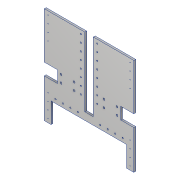
# Autodesk Inventor part: Piv Pannel
Saved by Autodesk Inventor 2018 (Build 220112000, 112)
## iProperties
Created: 2018-01-09
Part Number: Piv Pannel
Material: Aluminum 6061
Document SubType Name: Modeling
Designer: dsayers
Density: 2.7 g/cm^3
Appearance: Aluminum - Flat
Mass: 1658.47 g
Surface Area: 2042.47 cm^2
Volume: 614.249 cm^3
Author: dsayers
Autodesk Inventor part; units mm, degrees
ref_plane "YZ Plane" through (0, 0, 0) normal (1, 0, 0) x (0, 1, 0)
ref_plane "XZ Plane" through (0, 0, 0) normal (0, 1, 0) x (-1, 0, 0)
ref_plane "XY Plane" through (0, 0, 0) normal (0, 0, 1) x (1, 0, 0)
sketch "Sketch1" plane through (0, 0, 0) normal (0, 0, 1) x (1, 0, 0)
  line L0 (0, 0) -> (304.8, 0)
  line L1 (304.8, 0) -> (304.8, 330.2)
  line L2 (304.8, 330.2) -> (0, 330.2)
  line L3 (0, 330.2) -> (0, 0)
  dimension "d0" = 304.8
  dimension "d1" = 330.2
  constraints: 8 end point, 2 parallel, 1 horizontal, 1 perpendicular
  measures "d0" distance of L1.end L2.end
  measures "d1" distance of L0.end L1.end
extrude "Extrusion1" add sketch "Sketch1" along normal blind 6.35
sketch "Sketch2" plane through (0, 0, 6.35) normal (0, 0, 1) x (1, 0, 0)
  circle A0 centre (57.0998, 139.7) radius 3.175 projected
  circle A1 centre (101.5498, 165.1) radius 3.175 projected
  circle A2 centre (203.2502, 139.7) radius 3.175 projected
  circle A3 centre (247.7002, 165.1) radius 3.175 projected
  circle A4 centre (203.2502, 165.1) radius 3.175 projected
  circle A5 centre (247.7002, 139.7) radius 3.175 projected
  circle A6 centre (101.5498, 139.7) radius 3.175 projected
  circle A7 centre (57.0998, 165.1) radius 3.175 projected
  line L0 (0, 132.2) -> (44.7998, 132.2) projected
  line L1 (44.7998, 132.2) -> (44.7998, 172.6) projected
  line L2 (44.7998, 172.6) -> (0, 172.6) projected
  line L3 (0, 330.2) -> (0, 172.6) projected
  line L4 (304.8, 330.2) -> (0, 330.2) projected
  line L5 (304.8, 172.6) -> (304.8, 330.2) projected
  line L6 (304.8, 172.6) -> (260.0002, 172.6) projected
  line L7 (260.0002, 172.6) -> (260.0002, 132.2) projected
  line L8 (260.0002, 132.2) -> (304.8, 132.2) projected
  line L9 (304.8, 120.65) -> (304.8, 132.2) projected
  line L10 (0, 0) -> (22.86, 0) projected
  line L11 (0, 132.2) -> (0, 0) projected
  line L12 (44.7998, 172.6) -> (0, 172.6)
  line L13 (0, 172.6) -> (0, 132.2)
  line L14 (0, 132.2) -> (44.7998, 132.2)
  line L15 (44.7998, 132.2) -> (44.7998, 172.6)
  line L16 (260.0002, 172.6) -> (304.8, 172.6)
  line L17 (304.8, 172.6) -> (304.8, 132.2)
  line L18 (304.8, 132.2) -> (260.0002, 132.2)
  line L19 (260.0002, 132.2) -> (260.0002, 172.6)
  circle A8 centre (12.7, 38.1) radius 0.889 projected
  circle A9 centre (12.7, 88.9) radius 0.889 projected
  circle A10 centre (12.7, 266.7) radius 0.889 projected
  circle A11 centre (12.7, 317.5) radius 0.889 projected
  circle A12 centre (12.7, 292.1) radius 0.889 projected
  circle A13 centre (12.7, 241.3) radius 0.889 projected
  circle A14 centre (12.7, 63.5) radius 0.889 projected
  circle A15 centre (12.7, 12.7) radius 0.889 projected
  circle A16 centre (292.1, 266.7) radius 0.889 projected
  circle A17 centre (292.1, 317.5) radius 0.889 projected
  circle A18 centre (292.1, 292.1) radius 0.889 projected
  circle A19 centre (292.1, 241.3) radius 0.889 projected
  circle A20 centre (124.5248, 317.5) radius 2.2479 projected
  circle A21 centre (124.5248, 292.1) radius 2.2479 projected
  circle A22 centre (180.2752, 266.7) radius 2.2479 projected
  circle A23 centre (124.5248, 241.3) radius 2.2479 projected
  circle A24 centre (124.5248, 215.9) radius 2.2479 projected
  circle A25 centre (180.2752, 190.5) radius 2.2479 projected
  circle A26 centre (124.5248, 165.1) radius 2.2479 projected
  circle A27 centre (180.2752, 139.7) radius 2.2479 projected
  circle A28 centre (124.5248, 139.7) radius 2.2479 projected
  circle A29 centre (180.2752, 165.1) radius 2.2479 projected
  circle A30 centre (124.5248, 190.5) radius 2.2479 projected
  circle A31 centre (180.2752, 215.9) radius 2.2479 projected
  circle A32 centre (180.2752, 241.3) radius 2.2479 projected
  circle A33 centre (124.5248, 266.7) radius 2.2479 projected
  circle A34 centre (180.2752, 292.1) radius 2.2479 projected
  circle A35 centre (180.2752, 317.5) radius 2.2479 projected
  line L20 (167.5752, 120.65) -> (167.5752, 215.9) projected
  line L21 (167.5752, 215.9) -> (137.2248, 215.9) projected
  line L22 (137.2248, 215.9) -> (137.2248, 120.65) projected
  line L23 (22.86, 120.65) -> (22.86, 0) projected
  line L24 (304.8, 120.65) -> (167.5752, 120.65) projected
  line L25 (137.2248, 120.65) -> (22.86, 120.65) projected
  constraints: 16 end point, 4 parallel, 2 horizontal, 2 perpendicular
extrude "Extrusion2" cut sketch "Sketch2" against normal blind 6.35 contours L13 L2 L1 L0 | L17 L8 L7 L6
sketch "Sketch3" plane through (0, 0, 6.35) normal (0, 0, 1) x (1, 0, 0)
  circle A0 centre (57.0998, 139.7) radius 3.175 projected
  circle A1 centre (101.5498, 165.1) radius 3.175 projected
  circle A2 centre (203.2502, 139.7) radius 3.175 projected
  circle A3 centre (247.7002, 165.1) radius 3.175 projected
  circle A4 centre (203.2502, 165.1) radius 3.175 projected
  circle A5 centre (247.7002, 139.7) radius 3.175 projected
  circle A6 centre (101.5498, 139.7) radius 3.175 projected
  circle A7 centre (57.0998, 165.1) radius 3.175 projected
  line L0 (0, 132.2) -> (44.7998, 132.2) projected
  line L1 (44.7998, 132.2) -> (44.7998, 172.6) projected
  line L2 (44.7998, 172.6) -> (0, 172.6) projected
  line L3 (0, 330.2) -> (0, 172.6) projected
  line L4 (304.8, 330.2) -> (0, 330.2) projected
  line L5 (304.8, 172.6) -> (304.8, 330.2) projected
  line L6 (304.8, 172.6) -> (260.0002, 172.6) projected
  line L7 (260.0002, 172.6) -> (260.0002, 132.2) projected
  line L8 (260.0002, 132.2) -> (304.8, 132.2) projected
  line L9 (304.8, 120.65) -> (304.8, 132.2) projected
  line L10 (0, 0) -> (22.86, 0) projected
  line L11 (0, 132.2) -> (0, 0) projected
  circle A8 centre (12.7, 38.1) radius 0.889 projected
  circle A9 centre (12.7, 88.9) radius 0.889 projected
  circle A10 centre (12.7, 266.7) radius 0.889 projected
  circle A11 centre (12.7, 317.5) radius 0.889 projected
  circle A12 centre (12.7, 292.1) radius 0.889 projected
  circle A13 centre (12.7, 241.3) radius 0.889 projected
  circle A14 centre (12.7, 63.5) radius 0.889 projected
  circle A15 centre (12.7, 12.7) radius 0.889 projected
  circle A16 centre (292.1, 266.7) radius 0.889 projected
  circle A17 centre (292.1, 317.5) radius 0.889 projected
  circle A18 centre (292.1, 292.1) radius 0.889 projected
  circle A19 centre (292.1, 241.3) radius 0.889 projected
  circle A20 centre (124.5248, 317.5) radius 2.2479 projected
  circle A21 centre (124.5248, 292.1) radius 2.2479 projected
  circle A22 centre (180.2752, 266.7) radius 2.2479 projected
  circle A23 centre (124.5248, 241.3) radius 2.2479 projected
  circle A24 centre (124.5248, 215.9) radius 2.2479 projected
  circle A25 centre (180.2752, 190.5) radius 2.2479 projected
  circle A26 centre (124.5248, 165.1) radius 2.2479 projected
  circle A27 centre (180.2752, 139.7) radius 2.2479 projected
  circle A28 centre (124.5248, 139.7) radius 2.2479 projected
  circle A29 centre (180.2752, 165.1) radius 2.2479 projected
  circle A30 centre (124.5248, 190.5) radius 2.2479 projected
  circle A31 centre (180.2752, 215.9) radius 2.2479 projected
  circle A32 centre (180.2752, 241.3) radius 2.2479 projected
  circle A33 centre (124.5248, 266.7) radius 2.2479 projected
  circle A34 centre (180.2752, 292.1) radius 2.2479 projected
  circle A35 centre (180.2752, 317.5) radius 2.2479 projected
  line L12 (167.5752, 120.65) -> (167.5752, 215.9) projected
  line L13 (167.5752, 215.9) -> (137.2248, 215.9) projected
  line L14 (137.2248, 215.9) -> (137.2248, 120.65) projected
  line L15 (22.86, 120.65) -> (22.86, 0) projected
  line L16 (304.8, 120.65) -> (167.5752, 120.65) projected
  line L17 (137.2248, 120.65) -> (22.86, 120.65) projected
  point P0 (57.0998, 165.1)
  point P1 (57.0998, 139.7)
  point P2 (101.5498, 139.7)
  point P3 (101.5498, 165.1)
  point P4 (203.2502, 165.1)
  point P5 (203.2502, 139.7)
  point P6 (247.7002, 139.7)
  point P7 (247.7002, 165.1)
  constraints: 8 coincident
hole "Hole1" at (57.0998, 165.1, 6.35) at (57.0998, 139.7, 6.35) at (101.5498, 139.7, 6.35) at (101.5498, 165.1, 6.35) at (203.2502, 165.1, 6.35) at (203.2502, 139.7, 6.35) at (247.7002, 139.7, 6.35) at (247.7002, 165.1, 6.35) direction (0, 0, -1) diameter 6.35 depth 25.4 tip angle 118
sketch "Sketch4" plane through (0, 0, 6.35) normal (0, 0, 1) x (1, 0, 0)
  circle A0 centre (12.7, 38.1) radius 0.889 projected
  circle A1 centre (12.7, 88.9) radius 0.889 projected
  circle A2 centre (12.7, 266.7) radius 0.889 projected
  circle A3 centre (12.7, 317.5) radius 0.889 projected
  circle A4 centre (12.7, 292.1) radius 0.889 projected
  circle A5 centre (12.7, 241.3) radius 0.889 projected
  circle A6 centre (12.7, 63.5) radius 0.889 projected
  circle A7 centre (12.7, 12.7) radius 0.889 projected
  circle A8 centre (292.1, 266.7) radius 0.889 projected
  circle A9 centre (292.1, 317.5) radius 0.889 projected
  circle A10 centre (292.1, 292.1) radius 0.889 projected
  circle A11 centre (292.1, 241.3) radius 0.889 projected
  circle A12 centre (57.0998, 139.7) radius 3.175 projected
  circle A13 centre (101.5498, 165.1) radius 3.175 projected
  circle A14 centre (203.2502, 139.7) radius 3.175 projected
  circle A15 centre (247.7002, 165.1) radius 3.175 projected
  circle A16 centre (203.2502, 165.1) radius 3.175 projected
  circle A17 centre (247.7002, 139.7) radius 3.175 projected
  circle A18 centre (101.5498, 139.7) radius 3.175 projected
  circle A19 centre (57.0998, 165.1) radius 3.175 projected
  line L0 (0, 132.2) -> (44.7998, 132.2) projected
  line L1 (44.7998, 132.2) -> (44.7998, 172.6) projected
  line L2 (44.7998, 172.6) -> (0, 172.6) projected
  line L3 (0, 330.2) -> (0, 172.6) projected
  line L4 (304.8, 330.2) -> (0, 330.2) projected
  line L5 (304.8, 172.6) -> (304.8, 330.2) projected
  line L6 (304.8, 172.6) -> (260.0002, 172.6) projected
  line L7 (260.0002, 172.6) -> (260.0002, 132.2) projected
  line L8 (260.0002, 132.2) -> (304.8, 132.2) projected
  line L9 (304.8, 120.65) -> (304.8, 132.2) projected
  line L10 (0, 0) -> (22.86, 0) projected
  line L11 (0, 132.2) -> (0, 0) projected
  circle A20 centre (124.5248, 317.5) radius 2.2479 projected
  circle A21 centre (124.5248, 292.1) radius 2.2479 projected
  circle A22 centre (180.2752, 266.7) radius 2.2479 projected
  circle A23 centre (124.5248, 241.3) radius 2.2479 projected
  circle A24 centre (124.5248, 215.9) radius 2.2479 projected
  circle A25 centre (180.2752, 190.5) radius 2.2479 projected
  circle A26 centre (124.5248, 165.1) radius 2.2479 projected
  circle A27 centre (180.2752, 139.7) radius 2.2479 projected
  circle A28 centre (124.5248, 139.7) radius 2.2479 projected
  circle A29 centre (180.2752, 165.1) radius 2.2479 projected
  circle A30 centre (124.5248, 190.5) radius 2.2479 projected
  circle A31 centre (180.2752, 215.9) radius 2.2479 projected
  circle A32 centre (180.2752, 241.3) radius 2.2479 projected
  circle A33 centre (124.5248, 266.7) radius 2.2479 projected
  circle A34 centre (180.2752, 292.1) radius 2.2479 projected
  circle A35 centre (180.2752, 317.5) radius 2.2479 projected
  line L12 (167.5752, 120.65) -> (167.5752, 215.9) projected
  line L13 (167.5752, 215.9) -> (137.2248, 215.9) projected
  line L14 (137.2248, 215.9) -> (137.2248, 120.65) projected
  line L15 (22.86, 120.65) -> (22.86, 0) projected
  line L16 (304.8, 120.65) -> (167.5752, 120.65) projected
  line L17 (137.2248, 120.65) -> (22.86, 120.65) projected
  point P0 (12.7, 317.5)
  point P1 (12.7, 292.1)
  point P2 (12.7, 266.7)
  point P3 (12.7, 241.3)
  point P4 (12.7, 88.9)
  point P5 (292.1, 88.9)
  point P6 (292.1, 63.5)
  point P7 (292.1, 38.1)
  point P8 (292.1, 12.7)
  point P9 (292.1, 241.3)
  point P10 (292.1, 266.7)
  point P11 (292.1, 292.1)
  point P12 (292.1, 317.5)
  constraints: 12 coincident
hole "Hole2" at (12.7, 317.5, 6.35) at (12.7, 292.1, 6.35) at (12.7, 266.7, 6.35) at (12.7, 241.3, 6.35) at (12.7, 88.9, 6.35) at (12.7, 63.5, 6.35) at (12.7, 38.1, 6.35) at (12.7, 12.7, 6.35) at (292.1, 88.9, 6.35) at (292.1, 63.5, 6.35) at (292.1, 38.1, 6.35) at (292.1, 12.7, 6.35) at (292.1, 241.3, 6.35) at (292.1, 266.7, 6.35) at (292.1, 292.1, 6.35) at (292.1, 317.5, 6.35) direction (0, 0, -1) diameter 1.778 depth 25.4 tip angle 118 clearance for "Flat Head Machine Screw (82)" size "#0" standard "Ansi Unified Screw Threads"
sketch "Sketch5" plane through (0, 0, 6.35) normal (0, 0, 1) x (1, 0, 0)
  line L0 (165.1, 322.2478) -> (165.1, -126.1091) projected
  line L1 (139.7, 322.2478) -> (139.7, -126.1091) projected
  line L2 (139.7, 254) -> (165.1, 254)
  line L3 (165.1, 254) -> (165.1, 330.2)
  line L4 (165.1, 330.2) -> (139.7, 330.2)
  line L5 (139.7, 330.2) -> (139.7, 254)
  line L6 (304.8, 330.2) -> (0, 330.2) projected
  point P0 (0, 0)
  dimension "d20" = 0
  dimension "d21" = 76.2
  constraints: 8 end point, 2 parallel, 1 horizontal, 1 perpendicular, 1 point on line
  measures "d20" distance between parallel lines of L6 L4
  measures "d21" distance between parallel lines of L6 L2
extrude "Extrusion3" cut sketch "Sketch5" against normal blind 6.35
sketch "Sketch6" plane through (0, 0, 6.35) normal (0, 0, 1) x (1, 0, 0)
  line L0 (304.8, 330.2) -> (165.1, 330.2) projected
  line L1 (165.1, 330.2) -> (166.6875, 330.2)
  line L2 (166.6875, 330.2) -> (166.6875, 254)
  line L3 (166.6875, 254) -> (165.1, 254)
  line L4 (165.1, 254) -> (165.1, 330.2)
  line L5 (139.7, 330.2) -> (0, 330.2) projected
  line L6 (139.7, 330.2) -> (138.1125, 330.2)
  line L7 (138.1125, 330.2) -> (138.1125, 254)
  line L8 (138.1125, 254) -> (139.7, 254)
  line L9 (139.7, 254) -> (139.7, 330.2)
  line L10 (139.7, 254) -> (139.7, 330.2) projected
  point P0 (0, 0)
  dimension "d24" = 1.5875
  dimension "d25" = 1.5875
  constraints: 16 end point, 4 parallel, 2 horizontal, 2 perpendicular
  measures "d24" distance of L2.end L3.end
  measures "d25" distance between parallel lines of L10 L7
extrude "Extrusion4" cut sketch "Sketch6" against normal blind 6.35
sketch "Sketch7" plane through (0, 0, 6.35) normal (0, 0, 1) x (1, 0, 0)
  line L0 (142.24, 177.7506) -> (142.24, -148.2697) projected
  line L1 (165.1, 175.9057) -> (165.1, -141.7236) projected
  line L2 (139.7, 128.8943) -> (139.7, -188.735) projected
  line L3 (165.1, 175.9057) -> (139.7, 175.9057)
  line L4 (139.7, 175.9057) -> (139.7, 95.25)
  line L5 (139.7, 95.25) -> (165.1, 95.25)
  line L6 (165.1, 95.25) -> (165.1, 175.9057)
  line L7 (0, 0) -> (304.8, 0) projected
  line L8 (139.7, 175.9057) -> (165.1, 175.9057)
  line L9 (165.1, 175.9057) -> (165.1, 196.85)
  line L10 (165.1, 196.85) -> (139.7, 196.85)
  line L11 (139.7, 196.85) -> (139.7, 175.9057)
  dimension "d28" = 95.25
  dimension "d29" = 0
  dimension "d30" = 101.6
  constraints: 16 end point, 4 parallel, 2 horizontal, 2 perpendicular, 1 point on line
  measures "d28" distance between parallel lines of L7 L5
  measures "d29" distance between parallel lines of L1 L9
  measures "d30" distance between parallel lines of L5 L10
extrude "Extrusion5" cut sketch "Sketch7" against normal blind 6.35 contours L3 L1 L5 L0 | L3 L11 L10 L9 | L0 L5 L2 L4 L3
sketch "Sketch8" plane through (0, 0, 6.35) normal (0, 0, 1) x (1, 0, 0)
  line L0 (138.1125, 330.2) -> (138.1125, 254) projected
  line L1 (138.1125, 330.2) -> (166.6875, 330.2)
  line L2 (166.6875, 330.2) -> (166.6875, 95.25)
  line L3 (166.6875, 95.25) -> (138.1125, 95.25)
  line L4 (138.1125, 95.25) -> (138.1125, 330.2)
  line L5 (166.6875, 330.2) -> (166.6875, 254) projected
  line L6 (165.1, 95.25) -> (139.7, 95.25) projected
  point P0 (0, 0)
  dimension "d33" = 0
  dimension "d34" = 0
  constraints: 8 end point, 2 parallel, 1 horizontal, 1 perpendicular
  measures "d33" distance between parallel lines of L5 L2
  measures "d34" distance between parallel lines of L6 L3
extrude "Extrusion6" cut sketch "Sketch8" against normal blind 6.35
sketch "Sketch10" plane through (0, 0, 6.35) normal (0, 0, 1) x (1, 0, 0)
  circle A0 centre (124.5248, 317.5) radius 2.2479 projected
  circle A1 centre (124.5248, 292.1) radius 2.2479 projected
  circle A2 centre (180.2752, 266.7) radius 2.2479 projected
  circle A3 centre (124.5248, 241.3) radius 2.2479 projected
  circle A4 centre (124.5248, 215.9) radius 2.2479 projected
  circle A5 centre (180.2752, 190.5) radius 2.2479 projected
  circle A6 centre (124.5248, 165.1) radius 2.2479 projected
  circle A7 centre (180.2752, 139.7) radius 2.2479 projected
  circle A8 centre (124.5248, 139.7) radius 2.2479 projected
  circle A9 centre (180.2752, 165.1) radius 2.2479 projected
  circle A10 centre (124.5248, 190.5) radius 2.2479 projected
  circle A11 centre (180.2752, 215.9) radius 2.2479 projected
  circle A12 centre (180.2752, 241.3) radius 2.2479 projected
  circle A13 centre (124.5248, 266.7) radius 2.2479 projected
  circle A14 centre (180.2752, 292.1) radius 2.2479 projected
  circle A15 centre (180.2752, 317.5) radius 2.2479 projected
  circle A16 centre (12.7, 38.1) radius 0.889 projected
  circle A17 centre (12.7, 88.9) radius 0.889 projected
  circle A18 centre (12.7, 266.7) radius 0.889 projected
  circle A19 centre (12.7, 317.5) radius 0.889 projected
  circle A20 centre (12.7, 292.1) radius 0.889 projected
  circle A21 centre (12.7, 241.3) radius 0.889 projected
  circle A22 centre (12.7, 63.5) radius 0.889 projected
  circle A23 centre (12.7, 12.7) radius 0.889 projected
  circle A24 centre (292.1, 266.7) radius 0.889 projected
  circle A25 centre (292.1, 317.5) radius 0.889 projected
  circle A26 centre (292.1, 292.1) radius 0.889 projected
  circle A27 centre (292.1, 241.3) radius 0.889 projected
  circle A28 centre (57.0998, 139.7) radius 3.175 projected
  circle A29 centre (101.5498, 165.1) radius 3.175 projected
  circle A30 centre (203.2502, 139.7) radius 3.175 projected
  circle A31 centre (247.7002, 165.1) radius 3.175 projected
  circle A32 centre (203.2502, 165.1) radius 3.175 projected
  circle A33 centre (247.7002, 139.7) radius 3.175 projected
  circle A34 centre (101.5498, 139.7) radius 3.175 projected
  circle A35 centre (57.0998, 165.1) radius 3.175 projected
  line L0 (0, 132.2) -> (44.7998, 132.2) projected
  line L1 (44.7998, 132.2) -> (44.7998, 172.6) projected
  line L2 (44.7998, 172.6) -> (0, 172.6) projected
  line L3 (0, 330.2) -> (0, 172.6) projected
  line L4 (304.8, 330.2) -> (0, 330.2) projected
  line L5 (304.8, 172.6) -> (304.8, 330.2) projected
  line L6 (304.8, 172.6) -> (260.0002, 172.6) projected
  line L7 (260.0002, 172.6) -> (260.0002, 132.2) projected
  line L8 (260.0002, 132.2) -> (304.8, 132.2) projected
  line L9 (304.8, 120.65) -> (304.8, 132.2) projected
  line L10 (0, 0) -> (22.86, 0) projected
  line L11 (0, 132.2) -> (0, 0) projected
  line L12 (167.5752, 120.65) -> (167.5752, 215.9) projected
  line L13 (167.5752, 215.9) -> (137.2248, 215.9) projected
  line L14 (137.2248, 215.9) -> (137.2248, 120.65) projected
  line L15 (22.86, 120.65) -> (22.86, 0) projected
  line L16 (304.8, 120.65) -> (167.5752, 120.65) projected
  line L17 (137.2248, 120.65) -> (22.86, 120.65) projected
  constraints: 16 coincident
hole "Hole3" at (124.5248, 317.5, 6.35) at (124.5248, 292.1, 6.35) at (124.5248, 266.7, 6.35) at (124.5248, 241.3, 6.35) at (124.5248, 215.9, 6.35) at (124.5248, 190.5, 6.35) at (124.5248, 165.1, 6.35) at (124.5248, 139.7, 6.35) at (180.2752, 139.7, 6.35) at (180.2752, 165.1, 6.35) at (180.2752, 190.5, 6.35) at (180.2752, 215.9, 6.35) at (180.2752, 241.3, 6.35) at (180.2752, 266.7, 6.35) at (180.2752, 292.1, 6.35) at (180.2752, 317.5, 6.35) direction (0, 0, -1) diameter 4.4958 depth 25.4 tip angle 118 clearance for "Flat Head Machine Screw (82)" size "#8" standard "Ansi Unified Screw Threads"
sketch "Sketch11" plane through (0, 0, 0) normal (0, 0, -1) x (-1, 0, 0)
  line L0 (-22.86, 120.65) -> (-22.86, 0) projected
  line L1 (0, 0) -> (-22.86, 0) projected
  line L2 (0, 132.2) -> (0, 0) projected
  line L3 (0, 132.2) -> (-44.7998, 132.2) projected
  line L4 (-44.7998, 132.2) -> (-44.7998, 172.6) projected
  line L5 (-44.7998, 172.6) -> (0, 172.6) projected
  line L6 (0, 330.2) -> (0, 172.6) projected
  line L7 (-304.8, 330.2) -> (0, 330.2) projected
  line L8 (-304.8, 172.6) -> (-304.8, 330.2) projected
  line L9 (-304.8, 172.6) -> (-260.0002, 172.6) projected
  line L10 (-260.0002, 172.6) -> (-260.0002, 132.2) projected
  line L11 (-260.0002, 132.2) -> (-304.8, 132.2) projected
  line L12 (-304.8, 120.65) -> (-304.8, 132.2) projected
  line L13 (-304.8, 120.65) -> (-167.5752, 120.65) projected
  line L14 (-167.5752, 120.65) -> (-167.5752, 215.9) projected
  line L15 (-167.5752, 215.9) -> (-137.2248, 215.9) projected
  line L16 (-137.2248, 215.9) -> (-137.2248, 120.65) projected
  circle A0 centre (-124.5248, 317.5) radius 2.2479 projected
  circle A1 centre (-124.5248, 292.1) radius 2.2479 projected
  circle A2 centre (-180.2752, 266.7) radius 2.2479 projected
  circle A3 centre (-124.5248, 241.3) radius 2.2479 projected
  circle A4 centre (-124.5248, 215.9) radius 2.2479 projected
  circle A5 centre (-180.2752, 190.5) radius 2.2479 projected
  circle A6 centre (-124.5248, 165.1) radius 2.2479 projected
  circle A7 centre (-180.2752, 139.7) radius 2.2479 projected
  circle A8 centre (-124.5248, 139.7) radius 2.2479 projected
  circle A9 centre (-180.2752, 165.1) radius 2.2479 projected
  circle A10 centre (-124.5248, 190.5) radius 2.2479 projected
  circle A11 centre (-180.2752, 215.9) radius 2.2479 projected
  circle A12 centre (-180.2752, 241.3) radius 2.2479 projected
  circle A13 centre (-124.5248, 266.7) radius 2.2479 projected
  circle A14 centre (-180.2752, 292.1) radius 2.2479 projected
  circle A15 centre (-180.2752, 317.5) radius 2.2479 projected
  circle A16 centre (-12.7, 38.1) radius 0.889 projected
  circle A17 centre (-12.7, 88.9) radius 0.889 projected
  circle A18 centre (-12.7, 266.7) radius 0.889 projected
  circle A19 centre (-12.7, 317.5) radius 0.889 projected
  circle A20 centre (-12.7, 292.1) radius 0.889 projected
  circle A21 centre (-12.7, 241.3) radius 0.889 projected
  circle A22 centre (-12.7, 63.5) radius 0.889 projected
  circle A23 centre (-12.7, 12.7) radius 0.889 projected
  circle A24 centre (-292.1, 266.7) radius 0.889 projected
  circle A25 centre (-292.1, 317.5) radius 0.889 projected
  circle A26 centre (-292.1, 292.1) radius 0.889 projected
  circle A27 centre (-292.1, 241.3) radius 0.889 projected
  circle A28 centre (-57.0998, 139.7) radius 3.175 projected
  circle A29 centre (-101.5498, 165.1) radius 3.175 projected
  circle A30 centre (-203.2502, 139.7) radius 3.175 projected
  circle A31 centre (-247.7002, 165.1) radius 3.175 projected
  circle A32 centre (-203.2502, 165.1) radius 3.175 projected
  circle A33 centre (-247.7002, 139.7) radius 3.175 projected
  circle A34 centre (-101.5498, 139.7) radius 3.175 projected
  circle A35 centre (-57.0998, 165.1) radius 3.175 projected
  line L17 (-279.4, 69.85) -> (-22.86, 69.85)
  line L18 (-22.86, 69.85) -> (-22.86, 0)
  line L19 (-22.86, 0) -> (-279.4, 0)
  line L20 (-279.4, 0) -> (-279.4, 69.85)
  line L21 (-137.2248, 120.65) -> (-22.86, 120.65) projected
  constraints: 8 end point, 2 parallel, 1 horizontal, 1 perpendicular
extrude "Extrusion8" cut sketch "Sketch11" against normal blind 6.35 contours L0 L19 L20 L17
sketch "Sketch12" plane through (0, 0, 6.35) normal (0, 0, 1) x (1, 0, 0)
  line L0 (22.86, 120.65) -> (22.86, 0) projected
  line L1 (0, 0) -> (22.86, 0) projected
  line L2 (0, 132.2) -> (0, 0) projected
  line L3 (0, 132.2) -> (44.7998, 132.2) projected
  line L4 (44.7998, 132.2) -> (44.7998, 172.6) projected
  line L5 (44.7998, 172.6) -> (0, 172.6) projected
  line L6 (0, 330.2) -> (0, 172.6) projected
  line L7 (304.8, 330.2) -> (0, 330.2) projected
  line L8 (304.8, 172.6) -> (304.8, 330.2) projected
  line L9 (304.8, 172.6) -> (260.0002, 172.6) projected
  line L10 (260.0002, 172.6) -> (260.0002, 132.2) projected
  line L11 (260.0002, 132.2) -> (304.8, 132.2) projected
  line L12 (304.8, 120.65) -> (304.8, 132.2) projected
  line L13 (304.8, 120.65) -> (167.5752, 120.65) projected
  line L14 (167.5752, 120.65) -> (167.5752, 215.9) projected
  line L15 (167.5752, 215.9) -> (137.2248, 215.9) projected
  line L16 (137.2248, 215.9) -> (137.2248, 120.65) projected
  circle A0 centre (124.5248, 317.5) radius 2.2479 projected
  circle A1 centre (124.5248, 292.1) radius 2.2479 projected
  circle A2 centre (180.2752, 266.7) radius 2.2479 projected
  circle A3 centre (124.5248, 241.3) radius 2.2479 projected
  circle A4 centre (124.5248, 215.9) radius 2.2479 projected
  circle A5 centre (180.2752, 190.5) radius 2.2479 projected
  circle A6 centre (124.5248, 165.1) radius 2.2479 projected
  circle A7 centre (180.2752, 139.7) radius 2.2479 projected
  circle A8 centre (124.5248, 139.7) radius 2.2479 projected
  circle A9 centre (180.2752, 165.1) radius 2.2479 projected
  circle A10 centre (124.5248, 190.5) radius 2.2479 projected
  circle A11 centre (180.2752, 215.9) radius 2.2479 projected
  circle A12 centre (180.2752, 241.3) radius 2.2479 projected
  circle A13 centre (124.5248, 266.7) radius 2.2479 projected
  circle A14 centre (180.2752, 292.1) radius 2.2479 projected
  circle A15 centre (180.2752, 317.5) radius 2.2479 projected
  circle A16 centre (12.7, 38.1) radius 0.889 projected
  circle A17 centre (12.7, 88.9) radius 0.889 projected
  circle A18 centre (12.7, 266.7) radius 0.889 projected
  circle A19 centre (12.7, 317.5) radius 0.889 projected
  circle A20 centre (12.7, 292.1) radius 0.889 projected
  circle A21 centre (12.7, 241.3) radius 0.889 projected
  circle A22 centre (12.7, 63.5) radius 0.889 projected
  circle A23 centre (12.7, 12.7) radius 0.889 projected
  circle A24 centre (292.1, 266.7) radius 0.889 projected
  circle A25 centre (292.1, 317.5) radius 0.889 projected
  circle A26 centre (292.1, 292.1) radius 0.889 projected
  circle A27 centre (292.1, 241.3) radius 0.889 projected
  circle A28 centre (57.0998, 139.7) radius 3.175 projected
  circle A29 centre (101.5498, 165.1) radius 3.175 projected
  circle A30 centre (203.2502, 139.7) radius 3.175 projected
  circle A31 centre (247.7002, 165.1) radius 3.175 projected
  circle A32 centre (203.2502, 165.1) radius 3.175 projected
  circle A33 centre (247.7002, 139.7) radius 3.175 projected
  circle A34 centre (101.5498, 139.7) radius 3.175 projected
  circle A35 centre (57.0998, 165.1) radius 3.175 projected
  line L17 (137.2248, 120.65) -> (22.86, 120.65) projected
  point P0 (38.1, 82.55)
  point P1 (63.5, 82.55)
  point P2 (88.9, 82.55)
  point P3 (114.3, 82.55)
  point P4 (190.5, 82.55)
  point P5 (215.9, 82.55)
  point P6 (241.3, 82.55)
  point P7 (266.7, 82.55)
hole "Hole4" at (38.1, 82.55, 6.35) at (63.5, 82.55, 6.35) at (88.9, 82.55, 6.35) at (114.3, 82.55, 6.35) at (190.5, 82.55, 6.35) at (215.9, 82.55, 6.35) at (241.3, 82.55, 6.35) at (266.7, 82.55, 6.35) direction (0, 0, -1) diameter 4.4958 depth 25.4 tip angle 118 clearance for "Flat Head Machine Screw (82)" size "#8" standard "Ansi Unified Screw Threads"
body "Solid1"
